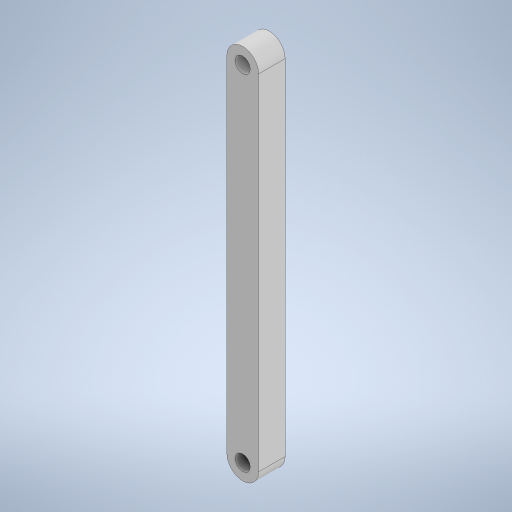
# Autodesk Inventor part: Exoskeleton 1
Saved by Autodesk Inventor 2023 (Build 270158000, 158)
## iProperties
Created: 2022-10-13
Part Number: Exoskeleton 1
Material: Generic
Document SubType Name: Modeling
Designer: GROS
Density: 1 g/cm^3
Appearance: Default
Author: GROS
Autodesk Inventor part; units mm, degrees
ref_plane "YZ Plane" through (0, 0, 0) normal (1, 0, 0) x (0, 1, 0)
ref_plane "XZ Plane" through (0, 0, 0) normal (0, 1, 0) x (-1, 0, 0)
ref_plane "XY Plane" through (0, 0, 0) normal (0, 0, 1) x (1, 0, 0)
sketch "Sketch1" plane through (0, 0, 0) normal (0, 0, 1) x (1, 0, 0)
  line L0 (0, 0) -> (6, 0)
  line L1 (6, 0) -> (6, 71)
  line L2 (6, 71) -> (0, 71)
  line L3 (0, 71) -> (0, 0)
  line L4 (3, 0) -> (3, 3)
  circle A0 centre (3, 3) radius 1.425
  circle A1 centre (3, 3) radius 3
  line L5 (3, 71) -> (3, 68)
  circle A2 centre (3, 68) radius 1.425
  circle A3 centre (3, 68) radius 3
  point P0 (6, 3)
  point P1 (6, 68)
  point P2 (0, 68)
  point P3 (0, 3)
  dimension "d10" = 6
  dimension "d11" = 71
  dimension "d12" = 3
  dimension "d13" = 6
  dimension "d14" = 2.85
  dimension "d15" = 3
  dimension "d16" = 6
  dimension "d17" = 2.85
  constraints: 12 end point, 4 centre point, 4 coincident, 2 midpoint, 2 parallel, 2 vertical, 1 horizontal, 1 perpendicular
  measures "d10" distance of L0.start L0.end
  measures "d11" distance of L2.end L0.start
  measures "d12" distance of L4.start L4.end
  measures "d13" diameter of A1
  measures "d14" diameter of A0
  measures "d15" distance of L5.start L5.end
  measures "d16" diameter of A3
  measures "d17" diameter of A2
extrude "Extrusion1" add sketch "Sketch1" along normal blind 5 contours A1 | L3 A3 L1 A1 | A3
body "Solid1"
